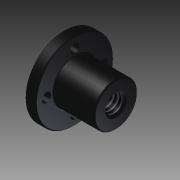
# Autodesk Inventor part: MTSRR10
Saved by Autodesk Inventor 2015 SP1 (Build 190203100, 203)
## iProperties
Category: PARTsolutions
Company: MISUMI
Created: 2015-02-02
Part Number: MTSRR10
Catalog Web Link: http://us.misumi-ec.com/vona2/detail/110300081660
Description: MTSRR-Nuts for 30 Degree Trapezoidal Screw Threads - High Load Flanged Resin Type - Round Flanged Type
Vendor: MISUMI
Document SubType Name: Modeling
Designer: PARTuser1
Manufacturer: MISUMI
Mass: 9.50204 g
Surface Area: 43.2585 cm^2
Volume: 9.50204 cm^3
Density: 1 g/cm^3
Material: Generic
Appearance: PSOLRGB-0-0-0
PSOL_IDENT_0: {\\10.0.0.236\data_v8\23d-libs\misumi\metric\10_lead_screws\mtsrr.prj},155 {VTYP=3D},{NB=MTSRR10},{L
PSOL_IDENT_1: INA=MTSRR10},{NN=MTSRR},{DATE=25.11.2014 11:59:53},{GEOMDATE=25.11.2014 00:00:00},{VERSION=},{LINEID=
PSOL_IDENT_2: 10},{LINESUBID=-1},{WBVAR=}  {NB=MTSRR10},{LINA=MTSRR10},{KT=DUMMY},{PN=MTSRR10},{MAT=PPS Resin with
PSOL_IDENT_3: Sliding Property (PTFE + GF30percent)},{OT=-45~200},{DD=10},{P=2},{D=20},{L1=24},{D1=36},{T=5},{PCD=
PSOL_IDENT_4: 26},{K=4.3},{ADT=278},{MASS=19}
SUPPLIER: MISUMI
ARTICLENO: MTSRR10
BOMINFO: MTSRR10
CREATOR: CADENAS GmbH
Title: MTSRR10
Author: Cadenas PARTsolutions
Comments: Nuts for 30 Degree Trapezoidal Screw Threads - High Load Flanged Resin Type - Round Flanged Type
Autodesk Inventor part; units mm, degrees
ref_plane "YZ Plane" through (0, 0, 0) normal (1, 0, 0) x (0, 1, 0)
ref_plane "XZ Plane" through (0, 0, 0) normal (0, 1, 0) x (-1, 0, 0)
ref_plane "XY Plane" through (0, 0, 0) normal (0, 0, 1) x (1, 0, 0)
sketch "Sketch_1" plane through (0, 0, 0) normal (0, 0, 1) x (1, 0, 0)
  line L0 (24, 0) -> (0, 0)
  line L1 (0, 0) -> (0, 17.5)
  line L2 (0, 17.5) -> (0.5, 18)
  line L3 (0.5, 18) -> (4.5, 18)
  line L4 (4.5, 18) -> (5, 17.5)
  line L5 (5, 17.5) -> (5, 10.5)
  arc A0 (5, 10.5) -> (5.5, 10) centre (5.5, 10.5) ccw
  line L6 (5.5, 10) -> (23.5, 10)
  line L7 (23.5, 10) -> (24, 9.5)
  line L8 (24, 9.5) -> (24, 0)
  line L9 (24, 0) -> (0, 0)
  constraints: 20 end point, 2 point on circle, 1 centre point
revolve "Revolution1" add sketch "Sketch_1" angle 360 about axis through (24, 0, 0) along (1, 0, 0)
sketch "Sketch_2" plane through (0, 0, 0) normal (0, 0, 1) x (1, 0, 0)
  line L0 (24, 0) -> (0, 0)
  line L1 (0, 0) -> (0, 5)
  line L2 (0, 5) -> (1, 4)
  line L3 (1, 4) -> (23, 4)
  line L4 (23, 4) -> (24, 5)
  line L5 (24, 5) -> (24, 0)
  line L6 (24, 0) -> (0, 0)
  constraints: 14 end point
revolve "Revolution2" cut sketch "Sketch_2" angle 360 about axis through (24, 0, 0) along (1, 0, 0)
thread "Thread1" size "TR10x2" class "7H" standard "ISO Metric Trapezoidal Threads" full length
sketch "Sketch_3" plane through (0, 0, 0) normal (0, 0, 1) x (1, 0, 0)
  line L0 (5, 13) -> (0, 13)
  line L1 (0, 13) -> (0, 15.15)
  line L2 (0, 15.15) -> (5, 15.15)
  line L3 (5, 15.15) -> (5, 13)
  line L4 (5, 13) -> (0, 13)
  constraints: 10 end point
revolve "Revolution3" cut sketch "Sketch_3" angle 360 about axis through (5, 13, 0) along (1, 0, 0)
pattern_linear "Rectangular Pattern1" count 2 spacing 18.3848 along (0, -0.7071, 0.7071) count 2 spacing 18.3848 along (0, -0.7071, -0.7071) of "Revolution3"
body "Solid1"
